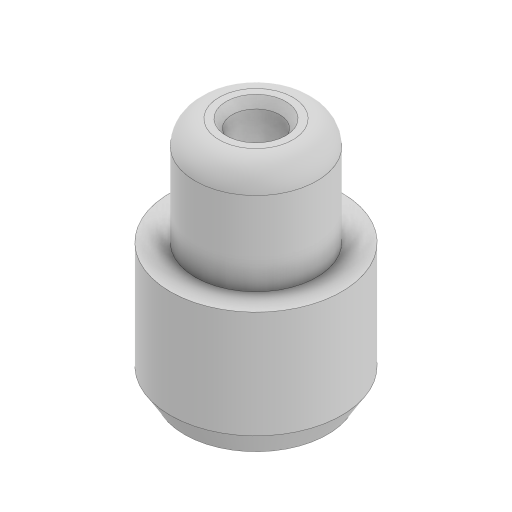
# Autodesk Inventor part: stylus_nib_base
Saved by Autodesk Inventor 2023 (Build 270158000, 158)
## iProperties
Created: 2023-03-26
Part Number: stylus_nib_base
Material: Generic
Document SubType Name: Modeling
Designer: James
Density: 1 g/cm^3
Appearance: Default
Author: James
## iProperties of the stored document stylus_nib_base_3DPrint.ipt
Created: 2023-04-01
Part Number: stylus_nib_base_3DPrint
Material: Generic
Document SubType Name: Modeling
Designer: James
Density: 1 g/cm^3
Appearance: Default
Author: James
## iProperties of the stored document MemberDocs/xDz0nufcfDcfpnyz54pdlkulfBg
Created: 2023-03-26
Part Number: stylus_nib_base
Material: Generic
Document SubType Name: Modeling
Designer: James
Density: 1 g/cm^3
Appearance: Default
Author: James
## iProperties of the stored document MemberDocs/x530fbnlcMk1r1cjd3qa1pbn4Th
Created: 2023-03-26
Part Number: stylus_nib_base
Material: Generic
Document SubType Name: Modeling
Designer: James
Density: 1 g/cm^3
Appearance: Default
Author: James
## iProperties of the stored document MemberDocs/xIv5z0e42GkwunkvaQ5jb2w0rPa
Created: 2023-03-26
Part Number: stylus_nib_base
Material: Generic
Document SubType Name: Modeling
Designer: James
Density: 1 g/cm^3
Appearance: Default
Author: James
## iProperties of the stored document MemberDocs/xE2o0nno0Akqa2cedByh3rzvnCa
Created: 2023-03-26
Part Number: stylus_nib_base
Material: Generic
Document SubType Name: Modeling
Designer: James
Density: 1 g/cm^3
Appearance: Default
Author: James
## iProperties of the stored document MemberDocs/xQiurgxpmK0tkpy5eR2jbirftXe
Created: 2023-03-26
Part Number: stylus_nib_base
Material: Generic
Document SubType Name: Modeling
Designer: James
Density: 1 g/cm^3
Appearance: Default
Author: James
## iProperties of the stored document MemberDocs/xQxcigsj0B0g5erx12kczo4quMe
Created: 2023-03-26
Part Number: stylus_nib_base
Material: Generic
Document SubType Name: Modeling
Designer: James
Density: 1 g/cm^3
Appearance: Default
Author: James
Autodesk Inventor part; units mm, degrees
ref_plane "YZ Plane" through (0, 0, 0) normal (1, 0, 0) x (0, 1, 0)
ref_plane "XZ Plane" through (0, 0, 0) normal (0, 1, 0) x (-1, 0, 0)
ref_plane "XY Plane" through (0, 0, 0) normal (0, 0, 1) x (1, 0, 0)
sketch "Sketch3" plane through (0, 0, 0) normal (1, 0, 0) x (0, 1, 0)
  line L0 (0, 0) -> (0, -3.6)
  line L1 (0, -3.6) -> (5.5, -3.6)
  line L2 (5.5, -3.6) -> (5.5, -2.55)
  line L3 (5.5, -2.55) -> (10, -2.55)
  line L4 (10, -2.55) -> (10, 0)
  line L5 (10, 0) -> (0, 0)
  dimension "baseRadius" = 3.6
  dimension "d12" = 10
  dimension "d13" = 2.55
  dimension "baseHeight" = 5.5
  constraints: 12 end point, 5 perpendicular, 1 vertical
  measures "baseRadius" distance of L0.start L0.end
  measures "d12" distance of L4.end L0.start
  measures "d13" distance of L3.end L4.end
  measures "baseHeight" distance of L0.end L1.end
revolve "Revolution1" add sketch "Sketch3" angle 360 about axis through (0, 10, 0) along (0, -1, 0)
sketch "Sketch4" plane through (0, 10, 0) normal (0, 1, 0) x (1, 0, 0)
  point P0 (0, 0)
hole "Hole2" at (0, 10, 0) direction (0, -1, 0) diameter 2 depth 6 countersink diameter 2.5 countersink angle 70
fillet "Fillet2" radius 1 1 edges at (0, 10, 2.55)
chamfer "Chamfer1" distance 0.6 distance2 1 1 edges at (0, 0, 3.6) measured on face at (0.7957, 0, -0.8982)
body "Solid1"
body "Solid2"
